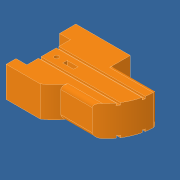
# Autodesk Inventor part: P1704_006
Saved by Autodesk Inventor 2019 (Build 230136000, 136)
## iProperties
Created: 2019-04-30
Part Number: P1704_006
Material: PLA
Document SubType Name: Modeling
Designer: Joan.MAILLARD
Density: 1.25 g/cm^3
Appearance: Orange
Project: P1704 Manette
Description: Gachette
Author: Joan.MAILLARD
Title: P1704_006_gachette
Autodesk Inventor part; units mm, degrees
ref_plane "YZ Plane" through (0, 0, 0) normal (1, 0, 0) x (0, 1, 0)
ref_plane "XZ Plane" through (0, 0, 0) normal (0, 1, 0) x (-1, 0, 0)
ref_plane "XY Plane" through (0, 0, 0) normal (0, 0, 1) x (1, 0, 0)
sketch "Esquisse2" plane through (0, 0, 0) normal (1, 0, 0) x (0, 1, 0)
  line L0 (-7, 10) -> (7, 10)
  line L1 (7, -10) -> (-7, -10)
  line L2 (-7, -10) -> (-7, 10)
  line L3 (-7, 10) -> (7, -10) construction
  line L4 (7, 10) -> (-7, -10) construction
  line L5 (7, -10) -> (7, 10)
  point P0 (0, 0)
  dimension "d2" = 20
  dimension "d7" = 14
  constraints: 12 end point, 2 midpoint, 2 parallel, 1 horizontal, 1 vertical
  measures "d2" distance of L1.end L0.start
  measures "d7" distance of L1.start L1.end
extrude "Extrusion1" add sketch "Esquisse2" along normal blind 20
sketch "Esquisse3" plane through (0, 0, 0) normal (-1, 0, 0) x (0, 0, 1)
  line L0 (-17.5, -7) -> (17.5, -7)
  line L1 (17.5, -7) -> (17.5, 7)
  line L2 (17.5, 7) -> (-17.5, 7)
  line L3 (-17.5, 7) -> (-17.5, -7)
  line L4 (-17.5, -7) -> (17.5, 7) construction
  line L5 (17.5, -7) -> (-17.5, 7) construction
  point P0 (0, 0)
  point P1 (-10, 7)
  dimension "d8" = 35
  constraints: 12 end point, 2 midpoint, 2 parallel, 1 horizontal, 1 perpendicular, 1 point on line
  measures "d8" distance between parallel lines of L1 L3
extrude "Extrusion2" add sketch "Esquisse3" along normal blind 25
sketch "Esquisse4" plane through (-25, 0, 0) normal (-1, 0, 0) x (0, 0, 1)
  line L0 (-10, -7) -> (-10, 7) projected
  line L1 (10, -7) -> (17.5, -7) projected
  line L2 (-10, 7) -> (10, 7)
  line L3 (10, 7) -> (10, -7)
  line L4 (10, -7) -> (-10, -7)
  line L5 (-10, -7) -> (-10, 7)
  point P0 (0, 0)
  constraints: 8 end point, 2 parallel, 1 horizontal, 1 perpendicular
extrude "Extrusion3" cut sketch "Esquisse4" against normal blind 5
sketch "Esquisse6" plane through (20, 7, 10) normal (0, 1, 0) x (1, 0, 0)
  line L0 (-20, -7.5) -> (-20, 0) construction
  line L1 (-40, 27.5) -> (-20, 27.5) construction
  line L2 (-20, 27.5) -> (-20, -7.5) construction
  line L3 (-20, -7.5) -> (-40, -7.5) construction
  line L4 (-40, -7.5) -> (-40, 27.5) construction
  line L5 (-40, 27.5) -> (-20, -7.5) construction
  line L6 (-20, 27.5) -> (-40, -7.5) construction
  line L7 (-32.5, 11) -> (-27.5, 11)
  line L8 (-27.5, 11) -> (-27.5, 9)
  line L9 (-27.5, 9) -> (-32.5, 9)
  line L10 (-32.5, 9) -> (-32.5, 11)
  line L11 (-32.5, 11) -> (-27.5, 9) construction
  line L12 (-27.5, 11) -> (-32.5, 9) construction
  point P0 (-20, 10)
  point P1 (-30, 10)
  point P2 (-40, 0)
  dimension "d15" = 2
  dimension "d16" = 5
  constraints: 24 end point, 4 midpoint, 4 parallel, 2 horizontal, 2 perpendicular, 1 coincident, 1 point on line
  measures "d15" distance of L7.end L8.end
  measures "d16" distance of L8.end L9.end
extrude "Extrusion6" cut sketch "Esquisse6" against normal blind 14
sketch "Esquisse8" plane through (-20, 0, 0) normal (-1, 0, 0) x (0, 0, 1)
  point P0 (0, 0)
  point P1 (0, 0)
  constraints: 1 coincident
hole "Perçage1" at (-20, 0, 0) direction (1, 0, 0) diameter 3 depth 12.5
sketch "Esquisse9" plane through (-25, 0, 0) normal (-1, 0, 0) x (0, 0, 1)
  line L0 (17.5, 7) -> (14.5, 7)
  line L1 (14.5, 7) -> (14.5, -7)
  line L2 (14.5, -7) -> (17.5, -7)
  line L3 (17.5, -7) -> (17.5, 7)
  line L4 (10, -7) -> (17.5, -7) projected
  dimension "d31" = 3
  constraints: 8 end point, 2 parallel, 1 coincident, 1 horizontal, 1 perpendicular, 1 point on line
  measures "d31" distance between parallel lines of L3 L1
extrude "Extrusion8" cut sketch "Esquisse9" against normal blind 20
fillet "Congé1" radius 2 6 edges at (20, 0, 10) (20, 0, -10) (10, 7, 10) (10, -7, 10) (10, 7, -10) (10, -7, -10)
sketch "Esquisse10" plane through (-25, 7, -17.5) normal (0, 1, 0) x (1, 0, 0)
  line L0 (12.5, -16.5) -> (5, -18.5) construction
  line L1 (5, -18.5) -> (5, -16.5) construction
  line L2 (5, -16.5) -> (12.5, -18.5) construction
  line L3 (12.5, -16.5) -> (17.5, -16.5) construction
  line L4 (17.5, -18.5) -> (12.5, -18.5) construction
  line L5 (5, -7.5) -> (5, -27.5) construction
  line L6 (12.5, -16.5) -> (12.5, -18.5) construction
  line L7 (12.5, -18.5) -> (12.5, -16.5) construction
  point P0 (25, -17.5)
  point P1 (8.75, -17.5)
  constraints: 8 end point, 2 equal length, 2 midpoint, 2 vertical, 1 point on line
hole "Perçage2" at (-16.25, 7, 0) direction (0, -1, 0) diameter 2 end through all
sketch "Esquisse11" plane through (-25, -7, -17.5) normal (0, -1, 0) x (1, 0, 0)
  line L0 (25, 27.5) -> (20.6125, 27.5)
  line L1 (25, 25.5) -> (25, 35) projected
  line L2 (20, 35) -> (20, 32) projected
  line L3 (43, 27.5) -> (25, 27.5) projected
  line L4 (0, 27.5) -> (0, 32) projected
  line L5 (25, 35) -> (20, 35) projected
  line L6 (0, 35) -> (25, 35)
  line L7 (5, 27.5) -> (5, 36.9505) construction
  arc A0 (20.6125, 27.5) -> (5, 35) centre (5, 15) ccw
  point P0 (25, 17.5)
  dimension "d55" = 20
  constraints: 6 end point, 6 point on line, 2 point on circle, 1 centre point, 1 coincident, 1 collinear, 1 horizontal, 1 tangent, 1 vertical
  measures "d55" radius of A0
extrude "Extrusion9" cut sketch "Esquisse11" against normal blind 14
sketch "Esquisse12" plane through (-25, -7, -17.5) normal (0, -1, 0) x (1, 0, 0)
  arc A0 (45, 9.5) -> (35, 27.5) centre (23.0044, 9.058) ccw
  line L0 (35, 27.5) -> (45, 27.5)
  line L1 (25, 25.5) -> (25, 27.5) projected
  line L2 (45, 27.5) -> (45, 9.5)
  line L3 (43, 27.5) -> (25, 27.5) projected
  point P0 (25, 17.5)
  dimension "d51" = 10
  dimension "d54" = 22
  constraints: 4 end point, 3 point on circle, 1 centre point, 1 horizontal, 1 point on line, 1 vertical
  measures "d51" distance from line of L0.start L1
  measures "d54" radius of A0
extrude "Extrusion10" cut sketch "Esquisse12" against normal blind 14
fillet "Congé3" radius 2 2 edges at (-2.1938, -7, 10) (-2.1938, 7, 10)
sketch "Esquisse13" plane through (-25, -7, -17.5) normal (0, -1, 0) x (1, 0, 0)
  line L0 (5, 22.2) -> (41.4812, 22.2)
  line L1 (41.4812, 22.2) -> (41.4812, 21)
  line L2 (41.4812, 21) -> (5, 21)
  line L3 (5, 21) -> (5, 22.2)
  arc A0 (45, 9.5) -> (37.6216, 25.5) centre (23.0044, 9.058) ccw projected
  line L4 (5, 27.5) -> (5, 7.5) projected
  line L5 (12.5, 18.5) -> (17.5, 18.5) projected
  line L6 (44.6839, 12.8) -> (5, 12.8)
  line L7 (5, 12.8) -> (5, 14)
  line L8 (5, 14) -> (44.6839, 14)
  line L9 (44.6839, 14) -> (44.6839, 12.8)
  line L10 (17.5, 16.5) -> (12.5, 16.5) projected
  point P0 (25, 17.5)
  dimension "d56" = 1.2
  dimension "d57" = 2.5
  dimension "d58" = 1.2
  dimension "d59" = 2.5
  constraints: 16 end point, 4 parallel, 2 horizontal, 2 perpendicular, 2 point on circle, 2 point on line
  measures "d56" distance between parallel lines of L2 L0
  measures "d57" distance between parallel lines of L2 L5
  measures "d58" distance between parallel lines of L6 L8
  measures "d59" distance between parallel lines of L8 L10
extrude "Extrusion11" cut sketch "Esquisse13" against normal blind 1 contours L0 A0 L2 L3 | L0 L1 A0 | L8 A0 L6 L4 | L8 L9 A0
sketch "Esquisse14" plane through (-25, 7, -17.5) normal (0, 1, 0) x (1, 0, 0)
  line L0 (5, -12.8) -> (44.6839, -12.8)
  line L1 (44.6839, -12.8) -> (44.6839, -14)
  line L2 (44.6839, -14) -> (5, -14)
  line L3 (5, -14) -> (5, -12.8)
  line L4 (5, -21) -> (41.4812, -21)
  line L5 (41.4812, -21) -> (41.4812, -22.2)
  line L6 (41.4812, -22.2) -> (5, -22.2)
  line L7 (5, -22.2) -> (5, -21)
  line L8 (44.6839, -12.8) -> (5, -12.8) projected
  arc A0 (37.6216, -25.5) -> (45, -9.5) centre (23.0044, -9.058) ccw projected
  line L9 (41.4812, -21) -> (5, -21) projected
  line L10 (5, -7.5) -> (5, -27.5) projected
  point P0 (25, -17.5)
  point P1 (44.4422, -14)
  point P2 (40.6478, -22.2)
  constraints: 16 end point, 4 parallel, 4 point on line, 2 horizontal, 2 perpendicular, 1 point on circle
extrude "Extrusion12" cut sketch "Esquisse14" against normal blind 1 contours L0 A0 L2 L3 | L1 L2 A0 | L4 A0 L6 L7 | L5 L6 A0
equation "\"d58\" = d56"
equation "\"d59\" = d57"
